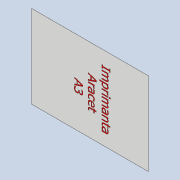
# Autodesk Inventor part: Foaie A3
Saved by Autodesk Inventor 2020 (Build 240168000, 168)
## iProperties
Created: 2021-02-20
Part Number: Foaie A3
Material: Generic
Document SubType Name: Modeling
Designer: Iulian Bors
Density: 1 g/cm^3
Appearance: Default
Author: Iulian Bors
Autodesk Inventor part; units mm, degrees
ref_plane "YZ Plane" through (0, 0, 0) normal (1, 0, 0) x (0, 1, 0)
ref_plane "XZ Plane" through (0, 0, 0) normal (0, 1, 0) x (-1, 0, 0)
ref_plane "XY Plane" through (0, 0, 0) normal (0, 0, 1) x (1, 0, 0)
sketch "Sketch1" plane through (0, 0, 0) normal (0, 0, 1) x (1, 0, 0)
  line L0 (-210, 148.5) -> (210, 148.5)
  line L1 (210, 148.5) -> (210, -148.5)
  line L2 (210, -148.5) -> (-210, -148.5)
  line L3 (-210, -148.5) -> (-210, 148.5)
  point P0 (0, 0)
  point P1 (0, 148.5)
  point P2 (-210, 0)
  dimension "d0" = 420
  dimension "d1" = 297
  constraints: 8 end point, 2 midpoint, 2 parallel, 1 horizontal, 1 horizontal alignment, 1 perpendicular, 1 vertical alignment
  measures "d0" distance of L0.start L0.end
  measures "d1" distance of L2.end L0.start
extrude "Extrusion1" add sketch "Sketch1" along normal blind 0.15
sketch "Sketch2" plane through (0, 0, 0.15) normal (0, 0, 1) x (1, 0, 0)
  line L0 (73.0273, 102.6897) -> (73.0273, 79.8495) construction
  line L1 (73.0273, 79.8495) -> (59.8584, 79.8495) construction
  line L2 (59.8584, 79.8495) -> (59.8584, 102.6897) construction
  line L3 (59.8584, 102.6897) -> (73.0273, 102.6897) construction
  line L4 (210, 148.5) -> (-210, 148.5) projected
  line L5 (42.8328, 89.197) -> (42.8328, 100.8177)
  line L6 (42.8328, 100.8177) -> (45.896, 100.8177)
  line L7 (45.896, 100.8177) -> (45.896, 97.0009)
  line L8 (45.896, 97.0009) -> (69.7696, 97.0009)
  line L9 (69.7696, 97.0009) -> (69.7696, 100.8177)
  line L10 (69.7696, 100.8177) -> (72.8328, 100.8177)
  line L11 (72.8328, 100.8177) -> (72.8328, 89.197)
  line L12 (72.8328, 89.197) -> (69.7696, 89.197)
  line L13 (69.7696, 89.197) -> (69.7696, 93.0139)
  line L14 (69.7696, 93.0139) -> (45.896, 93.0139)
  line L15 (45.896, 93.0139) -> (45.896, 89.197)
  line L16 (45.896, 89.197) -> (42.8328, 89.197)
  line L17 (42.8328, 59.0268) -> (55.8636, 59.0268)
  spline S0 degree 2 poles (55.8636, 59.0268) (57.4195, 59.0268) (60.0694, 59.2699) (60.7988, 59.6589) knots 0 0 0 1 2 2 2
  spline S1 degree 2 poles (60.7988, 59.6589) (61.601, 60.0479) (62.379, 61.5309) (62.379, 62.8194) knots 0 0 0 1 2 2 2
  spline S2 degree 2 poles (62.379, 62.8194) (62.379, 63.9863) (60.9446, 66.6605) (59.5832, 68.0706) knots 0 0 0 1 2 2 2
  spline S3 degree 2 poles (59.5832, 68.0706) (59.2429, 68.0463) (58.2947, 67.9976) (57.6626, 67.9976) knots 0 0 0 1 2 2 2
  line L18 (57.6626, 67.9976) -> (42.8328, 67.9976)
  line L19 (42.8328, 67.9976) -> (42.8328, 71.7902)
  line L20 (42.8328, 71.7902) -> (55.8636, 71.7902)
  spline S4 degree 2 poles (55.8636, 71.7902) (57.4195, 71.7902) (60.0694, 72.0333) (60.7988, 72.4223) knots 0 0 0 1 2 2 2
  spline S5 degree 2 poles (60.7988, 72.4223) (61.601, 72.8113) (62.379, 74.2942) (62.379, 75.5827) knots 0 0 0 1 2 2 2
  spline S6 degree 2 poles (62.379, 75.5827) (62.379, 76.7983) (60.8474, 79.4968) (59.6561, 80.761) knots 0 0 0 1 2 2 2
  line L21 (59.6561, 80.761) -> (42.8328, 80.761)
  line L22 (42.8328, 80.761) -> (42.8328, 84.5536)
  line L23 (42.8328, 84.5536) -> (65.345, 84.5536)
  line L24 (65.345, 84.5536) -> (65.345, 80.761)
  line L25 (65.345, 80.761) -> (62.8652, 80.761)
  spline S7 degree 2 poles (62.8652, 80.761) (64.3482, 79.278) (65.9771, 76.3607) (65.9771, 74.6103) knots 0 0 0 1 2 2 2
  spline S8 degree 2 poles (65.9771, 74.6103) (65.9771, 72.6168) (64.1537, 69.5292) (62.0873, 68.727) knots 0 0 0 1 2 2 2
  spline S9 degree 2 poles (62.0873, 68.727) (64.0078, 67.0009) (65.9771, 63.7432) (65.9771, 61.8469) knots 0 0 0 1 2 2 2
  spline S10 degree 2 poles (65.9771, 61.8469) (65.9771, 60.3882) (65.0775, 58.0057) (64.0565, 57.1305) knots 0 0 0 1 2 2 2
  spline S11 degree 2 poles (64.0565, 57.1305) (63.0354, 56.231) (59.9722, 55.2343) (57.6626, 55.2343) knots 0 0 0 1 2 2 2
  line L26 (57.6626, 55.2343) -> (42.8328, 55.2343)
  line L27 (42.8328, 55.2343) -> (42.8328, 59.0268)
  spline S12 degree 2 poles (54.6967, 31.0446) (49.0565, 31.0446) (42.3952, 36.4174) (42.3952, 40.526) knots 0 0 0 1 2 2 2
  spline S13 degree 2 poles (42.3952, 40.526) (42.3952, 42.2035) (43.1732, 44.7805) (43.9754, 46.1176) knots 0 0 0 1 2 2 2
  line L28 (43.9754, 46.1176) -> (34.5427, 46.1176)
  line L29 (34.5427, 46.1176) -> (34.5427, 49.9101)
  line L30 (34.5427, 49.9101) -> (65.345, 49.9101)
  line L31 (65.345, 49.9101) -> (65.345, 46.1176)
  line L32 (65.345, 46.1176) -> (62.9868, 46.1176)
  spline S14 degree 2 poles (62.9868, 46.1176) (64.2753, 44.7075) (65.9771, 41.2553) (65.9771, 39.2375) knots 0 0 0 1 2 2 2
  spline S15 degree 2 poles (65.9771, 39.2375) (65.9771, 35.372) (59.8506, 31.0446) (54.6967, 31.0446) knots 0 0 0 1 2 2 2
  spline S16 degree 2 poles (54.2591, 34.9587) (58.1245, 34.9587) (62.379, 37.4142) (62.379, 40.1613) knots 0 0 0 1 2 2 2
  spline S17 degree 2 poles (62.379, 40.1613) (62.379, 41.7659) (60.9446, 44.7805) (59.8263, 46.1176) knots 0 0 0 1 2 2 2
  line L33 (59.8263, 46.1176) -> (47.0386, 46.1176)
  spline S18 degree 2 poles (47.0386, 46.1176) (46.3336, 44.6346) (45.7988, 42.5195) (45.7988, 41.1581) knots 0 0 0 1 2 2 2
  spline S19 degree 2 poles (45.7988, 41.1581) (45.7988, 38.2164) (50.1262, 34.9587) (54.2591, 34.9587) knots 0 0 0 1 2 2 2
  line L34 (61.285, 15.1694) -> (61.285, 15.3639)
  spline S20 degree 2 poles (61.285, 15.3639) (61.4066, 15.8015) (61.4552, 16.7497) (61.4552, 17.4061) knots 0 0 0 1 2 2 2
  spline S21 degree 2 poles (61.4552, 17.4061) (61.4552, 18.9377) (60.1181, 21.9523) (58.8053, 23.3137) knots 0 0 0 1 2 2 2
  line L35 (58.8053, 23.3137) -> (42.8328, 23.3137)
  line L36 (42.8328, 23.3137) -> (42.8328, 27.1062)
  line L37 (42.8328, 27.1062) -> (65.345, 27.1062)
  line L38 (65.345, 27.1062) -> (65.345, 23.3137)
  line L39 (65.345, 23.3137) -> (61.99, 23.3137)
  spline S22 degree 2 poles (61.99, 23.3137) (63.8377, 21.2472) (65.345, 18.1597) (65.345, 16.701) knots 0 0 0 1 2 2 2
  spline S23 degree 2 poles (65.345, 16.701) (65.345, 16.1176) (65.2963, 15.5341) (65.2234, 15.1694) knots 0 0 0 1 2 2 2
  line L40 (65.2234, 15.1694) -> (61.285, 15.1694)
  line L41 (42.8328, 8.3623) -> (42.8328, 12.1549)
  line L42 (42.8328, 12.1549) -> (65.345, 12.1549)
  line L43 (65.345, 12.1549) -> (65.345, 8.3623)
  line L44 (65.345, 8.3623) -> (42.8328, 8.3623)
  line L45 (69.0889, 8.0949) -> (69.0889, 12.398)
  line L46 (69.0889, 12.398) -> (73.0273, 12.398)
  line L47 (73.0273, 12.398) -> (73.0273, 8.0949)
  line L48 (73.0273, 8.0949) -> (69.0889, 8.0949)
  line L49 (42.8328, -22.7317) -> (55.8636, -22.7317)
  spline S24 degree 2 poles (55.8636, -22.7317) (57.4195, -22.7317) (60.0694, -22.4886) (60.7988, -22.0996) knots 0 0 0 1 2 2 2
  spline S25 degree 2 poles (60.7988, -22.0996) (61.601, -21.7106) (62.379, -20.2276) (62.379, -18.9391) knots 0 0 0 1 2 2 2
  spline S26 degree 2 poles (62.379, -18.9391) (62.379, -17.7722) (60.9446, -15.098) (59.5832, -13.6879) knots 0 0 0 1 2 2 2
  spline S27 degree 2 poles (59.5832, -13.6879) (59.2429, -13.7122) (58.2947, -13.7609) (57.6626, -13.7609) knots 0 0 0 1 2 2 2
  line L50 (57.6626, -13.7609) -> (42.8328, -13.7609)
  line L51 (42.8328, -13.7609) -> (42.8328, -9.9683)
  line L52 (42.8328, -9.9683) -> (55.8636, -9.9683)
  spline S28 degree 2 poles (55.8636, -9.9683) (57.4195, -9.9683) (60.0694, -9.7252) (60.7988, -9.3362) knots 0 0 0 1 2 2 2
  spline S29 degree 2 poles (60.7988, -9.3362) (61.601, -8.9473) (62.379, -7.4643) (62.379, -6.1758) knots 0 0 0 1 2 2 2
  spline S30 degree 2 poles (62.379, -6.1758) (62.379, -4.9602) (60.8474, -2.2617) (59.6561, -0.9975) knots 0 0 0 1 2 2 2
  line L53 (59.6561, -0.9975) -> (42.8328, -0.9975)
  line L54 (42.8328, -0.9975) -> (42.8328, 2.795)
  line L55 (42.8328, 2.795) -> (65.345, 2.795)
  line L56 (65.345, 2.795) -> (65.345, -0.9975)
  line L57 (65.345, -0.9975) -> (62.8652, -0.9975)
  spline S31 degree 2 poles (62.8652, -0.9975) (64.3482, -2.4805) (65.9771, -5.3978) (65.9771, -7.1482) knots 0 0 0 1 2 2 2
  spline S32 degree 2 poles (65.9771, -7.1482) (65.9771, -9.1417) (64.1537, -12.2293) (62.0873, -13.0315) knots 0 0 0 1 2 2 2
  spline S33 degree 2 poles (62.0873, -13.0315) (64.0078, -14.7576) (65.9771, -18.0153) (65.9771, -19.9116) knots 0 0 0 1 2 2 2
  spline S34 degree 2 poles (65.9771, -19.9116) (65.9771, -21.3703) (65.0775, -23.7528) (64.0565, -24.628) knots 0 0 0 1 2 2 2
  spline S35 degree 2 poles (64.0565, -24.628) (63.0354, -25.5275) (59.9722, -26.5242) (57.6626, -26.5242) knots 0 0 0 1 2 2 2
  line L58 (57.6626, -26.5242) -> (42.8328, -26.5242)
  line L59 (42.8328, -26.5242) -> (42.8328, -22.7317)
  spline S36 degree 2 poles (45.2153, -44.393) (44.8749, -43.931) (43.6594, -42.3751) (43.2947, -41.6458) knots 0 0 0 1 2 2 2
  spline S37 degree 2 poles (43.2947, -41.6458) (42.7599, -40.649) (42.2007, -38.7771) (42.2007, -37.0753) knots 0 0 0 1 2 2 2
  spline S38 degree 2 poles (42.2007, -37.0753) (42.2007, -35.6896) (43.2461, -33.1855) (44.1942, -32.2374) knots 0 0 0 1 2 2 2
  spline S39 degree 2 poles (44.1942, -32.2374) (45.1181, -31.3379) (47.8409, -30.2438) (49.3482, -30.2438) knots 0 0 0 1 2 2 2
  spline S40 degree 2 poles (49.3482, -30.2438) (51.6821, -30.2438) (54.9884, -32.2131) (55.9365, -34.3524) knots 0 0 0 1 2 2 2
  spline S41 degree 2 poles (55.9365, -34.3524) (56.8117, -36.2487) (57.4681, -41.4027) (57.6383, -44.393) knots 0 0 0 1 2 2 2
  line L60 (57.6383, -44.393) -> (58.3677, -44.393)
  spline S42 degree 2 poles (58.3677, -44.393) (59.6805, -44.393) (61.3093, -43.5907) (61.7712, -42.8614) knots 0 0 0 1 2 2 2
  spline S43 degree 2 poles (61.7712, -42.8614) (62.2331, -42.132) (62.5249, -40.0413) (62.5249, -38.9229) knots 0 0 0 1 2 2 2
  spline S44 degree 2 poles (62.5249, -38.9229) (62.5249, -37.6101) (61.7469, -34.0607) (60.9933, -32.286) knots 0 0 0 1 2 2 2
  line L61 (60.9933, -32.286) -> (60.9933, -32.0672)
  line L62 (60.9933, -32.0672) -> (64.8587, -32.0672)
  spline S45 degree 2 poles (64.8587, -32.0672) (65.1505, -33.1126) (65.8798, -37.0267) (65.8798, -38.9473) knots 0 0 0 1 2 2 2
  spline S46 degree 2 poles (65.8798, -38.9473) (65.8798, -41.2811) (65.1505, -44.4659) (64.2023, -45.7301) knots 0 0 0 1 2 2 2
  spline S47 degree 2 poles (64.2023, -45.7301) (63.2785, -46.9699) (60.3369, -48.1855) (58.2218, -48.1855) knots 0 0 0 1 2 2 2
  line L63 (58.2218, -48.1855) -> (42.8328, -48.1855)
  line L64 (42.8328, -48.1855) -> (42.8328, -44.393)
  line L65 (42.8328, -44.393) -> (45.2153, -44.393)
  line L66 (48.3758, -44.393) -> (54.6237, -44.393)
  spline S48 degree 2 poles (54.6237, -44.393) (54.5022, -43.0315) (54.0889, -38.9229) (53.6999, -37.6344) knots 0 0 0 1 2 2 2
  spline S49 degree 2 poles (53.6999, -37.6344) (53.238, -36.1272) (51.3174, -34.1579) (49.6156, -34.1579) knots 0 0 0 1 2 2 2
  spline S50 degree 2 poles (49.6156, -34.1579) (47.6707, -34.1579) (45.7015, -36.346) (45.7015, -38.4367) knots 0 0 0 1 2 2 2
  spline S51 degree 2 poles (45.7015, -38.4367) (45.7015, -40.2114) (47.2331, -43.1288) (48.3758, -44.393) knots 0 0 0 1 2 2 2
  line L67 (42.8328, -71.1839) -> (42.8328, -67.3913)
  line L68 (42.8328, -67.3913) -> (55.6691, -67.3913)
  spline S52 degree 2 poles (55.6691, -67.3913) (57.225, -67.3913) (59.8993, -67.0996) (60.7015, -66.662) knots 0 0 0 1 2 2 2
  spline S53 degree 2 poles (60.7015, -66.662) (61.5524, -66.2001) (62.379, -64.5469) (62.379, -63.1369) knots 0 0 0 1 2 2 2
  spline S54 degree 2 poles (62.379, -63.1369) (62.379, -61.7268) (60.8717, -58.7366) (59.6561, -57.3022) knots 0 0 0 1 2 2 2
  line L69 (59.6561, -57.3022) -> (42.8328, -57.3022)
  line L70 (42.8328, -57.3022) -> (42.8328, -53.5097)
  line L71 (42.8328, -53.5097) -> (65.345, -53.5097)
  line L72 (65.345, -53.5097) -> (65.345, -57.3022)
  line L73 (65.345, -57.3022) -> (62.8409, -57.3022)
  spline S55 degree 2 poles (62.8409, -57.3022) (64.3725, -59.004) (65.9771, -62.286) (65.9771, -64.1336) knots 0 0 0 1 2 2 2
  spline S56 degree 2 poles (65.9771, -64.1336) (65.9771, -67.44) (61.601, -71.1839) (57.4438, -71.1839) knots 0 0 0 1 2 2 2
  line L74 (57.4438, -71.1839) -> (42.8328, -71.1839)
  spline S57 degree 2 poles (42.3952, -83.3152) (42.3952, -80.2276) (45.9203, -76.7511) (49.7372, -76.7511) knots 0 0 0 1 2 2 2
  line L75 (49.7372, -76.7511) -> (62.2088, -76.7511)
  line L76 (62.2088, -76.7511) -> (62.2088, -74.1985)
  line L77 (62.2088, -74.1985) -> (65.345, -74.1985)
  line L78 (65.345, -74.1985) -> (65.345, -76.7511)
  line L79 (65.345, -76.7511) -> (71.8117, -76.7511)
  line L80 (71.8117, -76.7511) -> (71.8117, -80.5437)
  line L81 (71.8117, -80.5437) -> (65.345, -80.5437)
  line L82 (65.345, -80.5437) -> (65.345, -87.521)
  line L83 (65.345, -87.521) -> (62.2088, -87.521)
  line L84 (62.2088, -87.521) -> (62.2088, -80.5437)
  line L85 (62.2088, -80.5437) -> (51.4876, -80.5437)
  spline S58 degree 2 poles (51.4876, -80.5437) (49.7858, -80.5437) (47.9138, -80.6652) (47.1116, -81.0785) knots 0 0 0 1 2 2 2
  spline S59 degree 2 poles (47.1116, -81.0785) (46.4066, -81.4189) (45.7015, -82.9505) (45.7015, -84.2633) knots 0 0 0 1 2 2 2
  spline S60 degree 2 poles (45.7015, -84.2633) (45.7015, -85.1871) (46.2607, -86.9132) (46.4309, -87.3022) knots 0 0 0 1 2 2 2
  line L86 (46.4309, -87.3022) -> (46.4309, -87.521)
  line L87 (46.4309, -87.521) -> (43.0273, -87.521)
  spline S61 degree 2 poles (43.0273, -87.521) (42.7356, -86.4513) (42.3952, -84.2633) (42.3952, -83.3152) knots 0 0 0 1 2 2 2
  spline S62 degree 2 poles (45.2153, -102.8614) (44.8749, -102.3994) (43.6594, -100.8435) (43.2947, -100.1142) knots 0 0 0 1 2 2 2
  spline S63 degree 2 poles (43.2947, -100.1142) (42.7599, -99.1174) (42.2007, -97.2455) (42.2007, -95.5437) knots 0 0 0 1 2 2 2
  spline S64 degree 2 poles (42.2007, -95.5437) (42.2007, -94.1579) (43.2461, -91.6539) (44.1942, -90.7058) knots 0 0 0 1 2 2 2
  spline S65 degree 2 poles (44.1942, -90.7058) (45.1181, -89.8062) (47.8409, -88.7122) (49.3482, -88.7122) knots 0 0 0 1 2 2 2
  spline S66 degree 2 poles (49.3482, -88.7122) (51.6821, -88.7122) (54.9884, -90.6814) (55.9365, -92.8208) knots 0 0 0 1 2 2 2
  spline S67 degree 2 poles (55.9365, -92.8208) (56.8117, -94.7171) (57.4681, -99.8711) (57.6383, -102.8614) knots 0 0 0 1 2 2 2
  line L88 (57.6383, -102.8614) -> (58.3677, -102.8614)
  spline S68 degree 2 poles (58.3677, -102.8614) (59.6805, -102.8614) (61.3093, -102.0591) (61.7712, -101.3297) knots 0 0 0 1 2 2 2
  spline S69 degree 2 poles (61.7712, -101.3297) (62.2331, -100.6004) (62.5249, -98.5097) (62.5249, -97.3913) knots 0 0 0 1 2 2 2
  spline S70 degree 2 poles (62.5249, -97.3913) (62.5249, -96.0785) (61.7469, -92.5291) (60.9933, -90.7544) knots 0 0 0 1 2 2 2
  line L89 (60.9933, -90.7544) -> (60.9933, -90.5356)
  line L90 (60.9933, -90.5356) -> (64.8587, -90.5356)
  spline S71 degree 2 poles (64.8587, -90.5356) (65.1505, -91.581) (65.8798, -95.4951) (65.8798, -97.4156) knots 0 0 0 1 2 2 2
  spline S72 degree 2 poles (65.8798, -97.4156) (65.8798, -99.7495) (65.1505, -102.9343) (64.2023, -104.1985) knots 0 0 0 1 2 2 2
  spline S73 degree 2 poles (64.2023, -104.1985) (63.2785, -105.4383) (60.3369, -106.6539) (58.2218, -106.6539) knots 0 0 0 1 2 2 2
  line L91 (58.2218, -106.6539) -> (42.8328, -106.6539)
  line L92 (42.8328, -106.6539) -> (42.8328, -102.8614)
  line L93 (42.8328, -102.8614) -> (45.2153, -102.8614)
  line L94 (48.3758, -102.8614) -> (54.6237, -102.8614)
  spline S74 degree 2 poles (54.6237, -102.8614) (54.5022, -101.4999) (54.0889, -97.3913) (53.6999, -96.1028) knots 0 0 0 1 2 2 2
  spline S75 degree 2 poles (53.6999, -96.1028) (53.238, -94.5955) (51.3174, -92.6263) (49.6156, -92.6263) knots 0 0 0 1 2 2 2
  spline S76 degree 2 poles (49.6156, -92.6263) (47.6707, -92.6263) (45.7015, -94.8144) (45.7015, -96.9051) knots 0 0 0 1 2 2 2
  spline S77 degree 2 poles (45.7015, -96.9051) (45.7015, -98.6798) (47.2331, -101.5972) (48.3758, -102.8614) knots 0 0 0 1 2 2 2
  line L95 (-6.5614, 51.3445) -> (23.4386, 41.231)
  line L96 (23.4386, 41.231) -> (23.4386, 36.3202)
  line L97 (23.4386, 36.3202) -> (-6.5614, 26.2067)
  line L98 (-6.5614, 26.2067) -> (-6.5614, 30.4126)
  line L99 (-6.5614, 30.4126) -> (1.826, 33.1354)
  line L100 (1.826, 33.1354) -> (1.826, 44.586)
  line L101 (1.826, 44.586) -> (-6.5614, 47.3088)
  line L102 (-6.5614, 47.3088) -> (-6.5614, 51.3445)
  line L103 (5.2295, 34.2294) -> (19.3543, 38.8728)
  line L104 (19.3543, 38.8728) -> (5.2295, 43.492)
  line L105 (5.2295, 43.492) -> (5.2295, 34.2294)
  line L106 (11.8908, 11.7173) -> (11.8908, 11.9117)
  spline S78 degree 2 poles (11.8908, 11.9117) (12.0123, 12.3493) (12.061, 13.2975) (12.061, 13.9539) knots 0 0 0 1 2 2 2
  spline S79 degree 2 poles (12.061, 13.9539) (12.061, 15.4855) (10.7238, 18.5001) (9.411, 19.8615) knots 0 0 0 1 2 2 2
  line L107 (9.411, 19.8615) -> (-6.5614, 19.8615)
  line L108 (-6.5614, 19.8615) -> (-6.5614, 23.654)
  line L109 (-6.5614, 23.654) -> (15.9508, 23.654)
  line L110 (15.9508, 23.654) -> (15.9508, 19.8615)
  line L111 (15.9508, 19.8615) -> (12.5958, 19.8615)
  spline S80 degree 2 poles (12.5958, 19.8615) (14.4435, 17.795) (15.9508, 14.7075) (15.9508, 13.2489) knots 0 0 0 1 2 2 2
  spline S81 degree 2 poles (15.9508, 13.2489) (15.9508, 12.6654) (15.9021, 12.0819) (15.8292, 11.7173) knots 0 0 0 1 2 2 2
  line L112 (15.8292, 11.7173) -> (11.8908, 11.7173)
  spline S82 degree 2 poles (-4.1789, -3.769) (-4.5193, -3.3071) (-5.7348, -1.7511) (-6.0995, -1.0218) knots 0 0 0 1 2 2 2
  spline S83 degree 2 poles (-6.0995, -1.0218) (-6.6343, -0.025) (-7.1935, 1.8469) (-7.1935, 3.5487) knots 0 0 0 1 2 2 2
  spline S84 degree 2 poles (-7.1935, 3.5487) (-7.1935, 4.9344) (-6.1481, 7.4385) (-5.2, 8.3866) knots 0 0 0 1 2 2 2
  spline S85 degree 2 poles (-5.2, 8.3866) (-4.2762, 9.2861) (-1.5533, 10.3801) (-0.046, 10.3801) knots 0 0 0 1 2 2 2
  spline S86 degree 2 poles (-0.046, 10.3801) (2.2879, 10.3801) (5.5942, 8.4109) (6.5423, 6.2715) knots 0 0 0 1 2 2 2
  spline S87 degree 2 poles (6.5423, 6.2715) (7.4175, 4.3753) (8.0739, -0.7787) (8.2441, -3.769) knots 0 0 0 1 2 2 2
  line L113 (8.2441, -3.769) -> (8.9734, -3.769)
  spline S88 degree 2 poles (8.9734, -3.769) (10.2862, -3.769) (11.9151, -2.9667) (12.377, -2.2374) knots 0 0 0 1 2 2 2
  spline S89 degree 2 poles (12.377, -2.2374) (12.8389, -1.508) (13.1307, 0.5827) (13.1307, 1.701) knots 0 0 0 1 2 2 2
  spline S90 degree 2 poles (13.1307, 1.701) (13.1307, 3.0139) (12.3527, 6.5633) (11.599, 8.338) knots 0 0 0 1 2 2 2
  line L114 (11.599, 8.338) -> (11.599, 8.5568)
  line L115 (11.599, 8.5568) -> (15.4645, 8.5568)
  spline S91 degree 2 poles (15.4645, 8.5568) (15.7563, 7.5114) (16.4856, 3.5973) (16.4856, 1.6767) knots 0 0 0 1 2 2 2
  spline S92 degree 2 poles (16.4856, 1.6767) (16.4856, -0.6571) (15.7563, -3.8419) (14.8081, -5.1061) knots 0 0 0 1 2 2 2
  spline S93 degree 2 poles (14.8081, -5.1061) (13.8843, -6.346) (10.9426, -7.5615) (8.8276, -7.5615) knots 0 0 0 1 2 2 2
  line L116 (8.8276, -7.5615) -> (-6.5614, -7.5615)
  line L117 (-6.5614, -7.5615) -> (-6.5614, -3.769)
  line L118 (-6.5614, -3.769) -> (-4.1789, -3.769)
  line L119 (-1.0185, -3.769) -> (5.2295, -3.769)
  spline S94 degree 2 poles (5.2295, -3.769) (5.108, -2.4075) (4.6947, 1.701) (4.3057, 2.9895) knots 0 0 0 1 2 2 2
  spline S95 degree 2 poles (4.3057, 2.9895) (3.8438, 4.4968) (1.9232, 6.466) (0.2214, 6.466) knots 0 0 0 1 2 2 2
  spline S96 degree 2 poles (0.2214, 6.466) (-1.7235, 6.466) (-3.6927, 4.278) (-3.6927, 2.1873) knots 0 0 0 1 2 2 2
  spline S97 degree 2 poles (-3.6927, 2.1873) (-3.6927, 0.4126) (-2.1611, -2.5048) (-1.0185, -3.769) knots 0 0 0 1 2 2 2
  spline S98 degree 2 poles (-7.0719, -21.8322) (-7.0719, -19.4983) (-5.6376, -15.6328) (-4.1789, -14.2471) knots 0 0 0 1 2 2 2
  spline S99 degree 2 poles (-4.1789, -14.2471) (-2.7445, -12.8614) (1.6801, -11.3297) (4.6461, -11.3297) knots 0 0 0 1 2 2 2
  spline S100 degree 2 poles (4.6461, -11.3297) (7.612, -11.3297) (11.9394, -12.91) (13.3981, -14.2471) knots 0 0 0 1 2 2 2
  spline S101 degree 2 poles (13.3981, -14.2471) (14.8811, -15.5842) (16.4613, -19.5469) (16.4613, -21.8322) knots 0 0 0 1 2 2 2
  spline S102 degree 2 poles (16.4613, -21.8322) (16.4613, -23.6798) (15.4159, -27.132) (14.7352, -28.4691) knots 0 0 0 1 2 2 2
  line L120 (14.7352, -28.4691) -> (10.4807, -28.4691)
  line L121 (10.4807, -28.4691) -> (10.4807, -28.2503)
  spline S103 degree 2 poles (10.4807, -28.2503) (10.8211, -27.837) (11.6963, -26.5729) (12.1582, -25.6733) knots 0 0 0 1 2 2 2
  spline S104 degree 2 poles (12.1582, -25.6733) (12.5472, -24.8711) (13.155, -22.7317) (13.155, -21.7592) knots 0 0 0 1 2 2 2
  spline S105 degree 2 poles (13.155, -21.7592) (13.155, -18.8176) (8.706, -15.2438) (4.6461, -15.2438) knots 0 0 0 1 2 2 2
  spline S106 degree 2 poles (4.6461, -15.2438) (0.6833, -15.2438) (-3.7656, -18.696) (-3.7656, -21.7592) knots 0 0 0 1 2 2 2
  spline S107 degree 2 poles (-3.7656, -21.7592) (-3.7656, -23.6069) (-2.234, -26.9618) (-1.0428, -28.2503) knots 0 0 0 1 2 2 2
  line L122 (-1.0428, -28.2503) -> (-1.0428, -28.4691)
  line L123 (-1.0428, -28.4691) -> (-5.2972, -28.4691)
  spline S108 degree 2 poles (-5.2972, -28.4691) (-5.5646, -27.91) (-6.3183, -26.2082) (-6.4885, -25.5275) knots 0 0 0 1 2 2 2
  spline S109 degree 2 poles (-6.4885, -25.5275) (-6.7802, -24.555) (-7.0719, -23.0234) (-7.0719, -21.8322) knots 0 0 0 1 2 2 2
  spline S110 degree 2 poles (-7.0719, -41.6944) (-7.0719, -36.2973) (-1.0185, -30.3654) (4.5731, -30.3654) knots 0 0 0 1 2 2 2
  spline S111 degree 2 poles (4.5731, -30.3654) (10.0674, -30.3654) (16.5828, -36.1272) (16.5828, -40.7706) knots 0 0 0 1 2 2 2
  spline S112 degree 2 poles (16.5828, -40.7706) (16.5828, -42.8614) (15.3673, -46.0947) (14.0788, -47.286) knots 0 0 0 1 2 2 2
  spline S113 degree 2 poles (14.0788, -47.286) (12.7903, -48.5015) (9.0707, -49.79) (6.3721, -49.79) knots 0 0 0 1 2 2 2
  line L124 (6.3721, -49.79) -> (4.3057, -49.79)
  line L125 (4.3057, -49.79) -> (4.3057, -34.2066)
  spline S114 degree 2 poles (4.3057, -34.2066) (0.3916, -34.2066) (-3.7656, -38.145) (-3.7656, -41.6458) knots 0 0 0 1 2 2 2
  spline S115 degree 2 poles (-3.7656, -41.6458) (-3.7656, -42.8857) (-3.2065, -45.2925) (-2.7689, -46.2649) knots 0 0 0 1 2 2 2
  spline S116 degree 2 poles (-2.7689, -46.2649) (-2.2826, -47.286) (-1.4317, -48.696) (-1.0428, -49.1579) knots 0 0 0 1 2 2 2
  line L126 (-1.0428, -49.1579) -> (-1.0428, -49.3767)
  line L127 (-1.0428, -49.3767) -> (-5.1757, -49.3767)
  spline S117 degree 2 poles (-5.1757, -49.3767) (-5.4431, -48.7203) (-6.221, -46.7268) (-6.4398, -45.9489) knots 0 0 0 1 2 2 2
  spline S118 degree 2 poles (-6.4398, -45.9489) (-6.7559, -44.8549) (-7.0719, -43.0558) (-7.0719, -41.6944) knots 0 0 0 1 2 2 2
  spline S119 degree 2 poles (7.1987, -46.0947) (8.7303, -46.0461) (10.967, -45.414) (11.7206, -44.8062) knots 0 0 0 1 2 2 2
  spline S120 degree 2 poles (11.7206, -44.8062) (12.5715, -44.1498) (13.471, -42.0834) (13.471, -40.5518) knots 0 0 0 1 2 2 2
  spline S121 degree 2 poles (13.471, -40.5518) (13.471, -39.0445) (12.5715, -36.9294) (11.6963, -36.0542) knots 0 0 0 1 2 2 2
  spline S122 degree 2 poles (11.6963, -36.0542) (10.7968, -35.2033) (8.6331, -34.3281) (7.1987, -34.2066) knots 0 0 0 1 2 2 2
  line L128 (7.1987, -34.2066) -> (7.1987, -46.0947)
  spline S123 degree 2 poles (-6.999, -60.4383) (-6.999, -57.3508) (-3.4739, -53.8743) (0.343, -53.8743) knots 0 0 0 1 2 2 2
  line L129 (0.343, -53.8743) -> (12.8146, -53.8743)
  line L130 (12.8146, -53.8743) -> (12.8146, -51.3216)
  line L131 (12.8146, -51.3216) -> (15.9508, -51.3216)
  line L132 (15.9508, -51.3216) -> (15.9508, -53.8743)
  line L133 (15.9508, -53.8743) -> (22.4175, -53.8743)
  line L134 (22.4175, -53.8743) -> (22.4175, -57.6669)
  line L135 (22.4175, -57.6669) -> (15.9508, -57.6669)
  line L136 (15.9508, -57.6669) -> (15.9508, -64.6442)
  line L137 (15.9508, -64.6442) -> (12.8146, -64.6442)
  line L138 (12.8146, -64.6442) -> (12.8146, -57.6669)
  line L139 (12.8146, -57.6669) -> (2.0934, -57.6669)
  spline S124 degree 2 poles (2.0934, -57.6669) (0.3916, -57.6669) (-1.4804, -57.7884) (-2.2826, -58.2017) knots 0 0 0 1 2 2 2
  spline S125 degree 2 poles (-2.2826, -58.2017) (-2.9877, -58.5421) (-3.6927, -60.0737) (-3.6927, -61.3865) knots 0 0 0 1 2 2 2
  spline S126 degree 2 poles (-3.6927, -61.3865) (-3.6927, -62.3103) (-3.1335, -64.0364) (-2.9633, -64.4254) knots 0 0 0 1 2 2 2
  line L140 (-2.9633, -64.4254) -> (-2.9633, -64.6442)
  line L141 (-2.9633, -64.6442) -> (-6.3669, -64.6442)
  spline S127 degree 2 poles (-6.3669, -64.6442) (-6.6586, -63.5745) (-6.999, -61.3865) (-6.999, -60.4383) knots 0 0 0 1 2 2 2
  line L142 (-55.9556, 12.6897) -> (-25.9556, 2.5762)
  line L143 (-25.9556, 2.5762) -> (-25.9556, -2.3346)
  line L144 (-25.9556, -2.3346) -> (-55.9556, -12.4481)
  line L145 (-55.9556, -12.4481) -> (-55.9556, -8.2422)
  line L146 (-55.9556, -8.2422) -> (-47.5683, -5.5194)
  line L147 (-47.5683, -5.5194) -> (-47.5683, 5.9312)
  line L148 (-47.5683, 5.9312) -> (-55.9556, 8.654)
  line L149 (-55.9556, 8.654) -> (-55.9556, 12.6897)
  line L150 (-44.1647, -4.4254) -> (-30.0399, 0.2181)
  line L151 (-30.0399, 0.2181) -> (-44.1647, 4.8372)
  line L152 (-44.1647, 4.8372) -> (-44.1647, -4.4254)
  spline S128 degree 2 poles (-28.8, -22.5372) (-28.8, -21.4432) (-29.3349, -19.2795) (-29.7482, -18.2341) knots 0 0 0 1 2 2 2
  spline S129 degree 2 poles (-29.7482, -18.2341) (-30.1615, -17.2617) (-31.0367, -15.8273) (-31.4256, -15.2682) knots 0 0 0 1 2 2 2
  line L153 (-31.4256, -15.2682) -> (-31.4256, -15.025)
  line L154 (-31.4256, -15.025) -> (-27.1712, -15.025)
  spline S130 degree 2 poles (-27.1712, -15.025) (-26.4662, -16.3379) (-25.3235, -20.8354) (-25.3235, -22.8532) knots 0 0 0 1 2 2 2
  spline S131 degree 2 poles (-25.3235, -22.8532) (-25.3235, -24.8954) (-26.1501, -27.9343) (-27.0253, -29.1742) knots 0 0 0 1 2 2 2
  spline S132 degree 2 poles (-27.0253, -29.1742) (-27.9734, -30.487) (-30.7206, -31.8484) (-32.5683, -31.8484) knots 0 0 0 1 2 2 2
  spline S133 degree 2 poles (-32.5683, -31.8484) (-35.048, -31.8484) (-38.7919, -28.5907) (-39.2781, -26.3054) knots 0 0 0 1 2 2 2
  line L155 (-39.2781, -26.3054) -> (-39.5699, -26.3054)
  spline S134 degree 2 poles (-39.5699, -26.3054) (-39.7644, -27.2536) (-40.6396, -29.4173) (-41.5148, -30.3411) knots 0 0 0 1 2 2 2
  spline S135 degree 2 poles (-41.5148, -30.3411) (-42.3657, -31.2649) (-45.0885, -32.4319) (-47.0577, -32.4319) knots 0 0 0 1 2 2 2
  spline S136 degree 2 poles (-47.0577, -32.4319) (-49.0756, -32.4319) (-52.5034, -31.0461) (-53.8162, -29.7819) knots 0 0 0 1 2 2 2
  spline S137 degree 2 poles (-53.8162, -29.7819) (-55.1777, -28.4691) (-56.5877, -24.7495) (-56.5877, -22.3913) knots 0 0 0 1 2 2 2
  spline S138 degree 2 poles (-56.5877, -22.3913) (-56.5877, -20.1304) (-55.4937, -15.7058) (-54.7401, -14.1985) knots 0 0 0 1 2 2 2
  line L156 (-54.7401, -14.1985) -> (-50.4856, -14.1985)
  line L157 (-50.4856, -14.1985) -> (-50.4856, -14.4902)
  spline S139 degree 2 poles (-50.4856, -14.4902) (-51.4094, -15.7544) (-53.1112, -20.0332) (-53.1112, -22.1482) knots 0 0 0 1 2 2 2
  spline S140 degree 2 poles (-53.1112, -22.1482) (-53.1112, -23.3881) (-52.3333, -25.8678) (-51.4337, -26.6944) knots 0 0 0 1 2 2 2
  spline S141 degree 2 poles (-51.4337, -26.6944) (-50.5342, -27.4967) (-48.3948, -28.3476) (-46.766, -28.3476) knots 0 0 0 1 2 2 2
  spline S142 degree 2 poles (-46.766, -28.3476) (-45.1371, -28.3476) (-43.0221, -27.3994) (-42.4143, -26.5485) knots 0 0 0 1 2 2 2
  spline S143 degree 2 poles (-42.4143, -26.5485) (-41.8065, -25.6977) (-41.3446, -23.3881) (-41.3446, -22.0267) knots 0 0 0 1 2 2 2
  line L158 (-41.3446, -22.0267) -> (-41.3446, -20.3249)
  line L159 (-41.3446, -20.3249) -> (-38.014, -20.3249)
  line L160 (-38.014, -20.3249) -> (-38.014, -21.662)
  spline S144 degree 2 poles (-38.014, -21.662) (-38.014, -24.3605) (-35.437, -27.7641) (-32.9815, -27.7641) knots 0 0 0 1 2 2 2
  spline S145 degree 2 poles (-32.9815, -27.7641) (-31.8389, -27.7641) (-30.2101, -26.8889) (-29.7239, -26.1839) knots 0 0 0 1 2 2 2
  spline S146 degree 2 poles (-29.7239, -26.1839) (-29.2133, -25.4302) (-28.8, -23.5826) (-28.8, -22.5372) knots 0 0 0 1 2 2 2
  point P0 (0, 0)
  constraints: 1 parallel, 2 other
extrude "Extrusion2" add sketch "Sketch2" along normal blind 0.01
body "Solid1"
